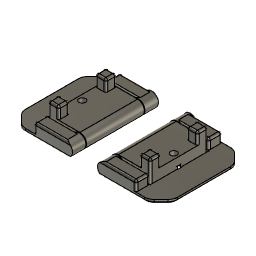
Voron-Simple-Hinge v20 (Autodesk Fusion 360 design; units mm, degrees)
Autodesk Fusion 360 part; units mm, degrees
note: some values were not read from the file. Set by a fixed rule: which sketch regions a step uses.
sketch "Sketch1" plane through (0, 0, 0) normal (0, 0, 1) x (1, 0, 0)
  circle A0 centre (0, 0) radius 1.6
  circle A1 centre (0, 0) radius 3.5
  line L0 (0, -3.5) -> (-16.5, -3.5)
  line L1 (-16.5, -3.5) -> (-16.5, 3.4)
  line L2 (-11, -3.5) -> (-11, -9.5)
  line L3 (-11, -9.5) -> (-16.5, -9.5)
  line L4 (-16.5, -9.5) -> (-16.5, -3.5)
  line L5 (-16.4, 3.5) -> (0, 3.5)
  arc A2 (-16.4, 3.5) -> (-16.5, 3.4) centre (-16.4, 3.4) ccw
  line L6 (-13.0173, 3.5) -> (-29.4, 3.5)
  line L7 (-29.5, 3.4) -> (-29.5, 1.5)
  line L8 (-29.5, 1.5) -> (-16.5, 1.5)
  arc A3 (-29.4, 3.5) -> (-29.5, 3.4) centre (-29.4, 3.4) ccw
  line L9 (-16.7917, 1.5) -> (-16.7917, 3.5)
  line L10 (0, 0) -> (-16.7917, 3.4812) construction
  line L11 (0, 0) -> (-16.7917, 2.5) construction
  line L12 (-3.5, 3.5) -> (-3.5, -3.5) construction
  line L13 (-29.5, 2.5) -> (-28.5, 3.5)
  line L14 (-16.5, 2.5) -> (-15.3897, 3.6103)
  line L15 (1.4497, 3.5) -> (2.4749, 2.4749)
  line L16 (0, 3.5) -> (1.4497, 3.5)
  point P0 (-16.5, 4.25)
  point P1 (-16.4979, 3.4203)
  dimension "d1" = 3.2
  dimension "d2" = 7
  dimension "d5" = 5.5
  dimension "d6" = 6
  dimension "d18" = 0.1
  dimension "d20" = 5
  dimension "d21" = 13
  dimension "d22" = 0.1
  dimension "d25" = 0.3
  dimension "d63" = 13
  dimension "d81" = 45
  dimension "d82" = 45
  dimension "d83" = 1
  dimension "d84" = 45
  constraint coincident A0.centre A1.centre
  constraint concentric A0 A1
  constraint horizontal L0
  constraint vertical L1
  constraint coincident A1 L0.start
  constraint tangent A1 L0
  constraint vertical L2
  constraint horizontal L3
  constraint vertical L4
  constraint coincident P0 L1
  constraint coincident A1 L5.end
  constraint tangent A1 L5
  constraint tangent L5 A2
  constraint tangent L1 A2
  constraint horizontal L5
  constraint horizontal L6
  constraint vertical L7
  constraint horizontal L8
  constraint coincident L5 L6.start
  constraint tangent L6 A3
  constraint tangent L7 A3
  constraint coincident L1 L8.end
  constraint coincident L8 L9.start
  constraint coincident L6 L9.end
  constraint perpendicular L6 L9
  constraint coincident L9 L10.end
  constraint coincident A2.centre L10
  constraint coincident A2 P1
  constraint coincident L10 P1
  constraint midpoint L9 L11.end
  constraint coincident L0 L2.start
  constraint coincident L5 L12.start
  constraint coincident L0 L12.end
  constraint perpendicular L0 L12
  constraint tangent A1 L12
  constraint coincident L7 L13.start
  constraint coincident L6 L13.end
  constraint coincident L1 L14.start
  constraint horizontal L13.start L14.start
  constraint coincident A1 L15.end
  constraint tangent A1 L15
  constraint coincident L15 L16.end
  constraint tangent A1 L16
  constraint coincident L15.start L16.end
  measures "d1" diameter of A0
  measures "d2" diameter of A1
  measures "d5" distance of L2.end L3.end
  measures "d6" distance of L0.end L3.end
  measures "d18" radius of A2
  measures "d20" distance of L0 L8
  measures "d21" distance of L1 L7
  measures "d22" radius of A3
  measures "d25" distance of L10.end P1
  measures "d63" distance of L1 L12
  measures "d81" angle of L7 L13
  measures "d82" angle of L1 L14
  measures "d83" distance of L6 L13.start
  measures "d84" angle of L15 L16
sketch "Sketch3" plane through (0, 0, 0) normal (0, 0, 1) x (1, 0, 0)
  circle A0 centre (0, 0) radius 2.35
  circle A1 centre (0, 0) radius 3.5
  dimension "d78" = 4.7
  constraint coincident A0.centre A1.centre
  measures "d78" diameter of A0
extrude "Extrude1" add sketch "Sketch1" along normal blind 5.5 contours A1 | A1 L15 L16 | A1 L0 L1 L5 L6 L14 | L0 L2 L3 L4 makes body 1
extrude "Extrude2" add sketch "Sketch1" along normal blind 19 from surface at 5.5 contours A1 | A1 L15 L16 | A1 L0 L1 L5 L6 L14 bodies 1
extrude "Extrude3" add sketch "Sketch1" along normal blind 5.5 from surface at 24.5 contours A1 | A1 L15 L16 | A1 L0 L1 L5 L6 L14 | L0 L2 L3 L4 bodies 1
extrude "Extrude4" add sketch "Sketch1" against normal blind 7 from surface at -0.3 separate body contours A0 | A1 | A1 L15 L16 | A1 L0 L1 L5 L6 L14 | L1 L5 A2 L6 L14 | L1 A2 L6 L8 L9 | L6 L7 L8 L9 L13 makes body 2
extrude "Extrude15" cut sketch "Sketch3" against normal up to surface (4.3 mm away) contours A0 bodies 2
extrude "Extrude5" add sketch "Sketch1" along normal up to surface (30.6 mm away) from surface at -0.3 contours L6 L7 L8 L9 L13 bodies 2
extrude "Extrude6" add sketch "Sketch1" along normal blind 7 from surface at 30.3 contours A1 | A1 L15 L16 | A1 L0 L1 L5 L6 L14 | L1 L5 A2 L6 L14 | L1 A2 L6 L8 L9 | L6 L7 L8 L9 L13 bodies 2
sketch "Sketch2" plane through (0, -3.5, 0) normal (0, -1, 0) x (1, 0, 0)
  line L0 (-11, 0) -> (0, 0)
  line L1 (0, 0) -> (0, 30)
  line L2 (0, 30) -> (-11, 30)
  line L3 (-11, 30) -> (-11, 24.5)
  line L4 (-11, 24.5) -> (-16.5, 24.5)
  line L5 (-16.5, 24.5) -> (-16.5, 5.5)
  line L6 (-16.5, 5.5) -> (-11, 5.5)
  line L7 (-11, 5.5) -> (-11, 0)
  line L8 (-13.75, 24.5) -> (-13.75, 5.5) construction
  circle A0 centre (-13.75, 15) radius 1.7
  circle A1 centre (-13.75, 15) radius 2.85
  line L9 (-29.5, 37.3) -> (-29.5, -7.3)
  line L10 (-29.5, -7.3) -> (-16.5, -7.3)
  line L11 (-16.5, -7.3) -> (-16.5, -0.3)
  line L12 (-16.5, -0.3) -> (-16.7917, -0.3)
  line L13 (-16.7917, -0.3) -> (-16.7917, 30.3)
  line L14 (-16.7917, 30.3) -> (-16.5, 30.3)
  line L15 (-16.5, 30.3) -> (-16.5, 37.3)
  line L16 (-16.5, 37.3) -> (-29.5, 37.3)
  line L17 (-23, 37.3) -> (-29.5, 30.8)
  line L18 (-13.75, 15) -> (-29.5, 15) construction
  line L19 (-23, -7.3) -> (-29.5, -0.8)
  circle A2 centre (-13.75, 15) radius 3.35
  dimension "d35" = 3.4
  dimension "d36" = 5.7
  dimension "d38" = 45
  dimension "d61" = 0.5
  constraint midpoint L4 L8.start
  constraint midpoint L6 L8.end
  constraint midpoint L8 A0.centre
  constraint concentric A0 A1
  constraint coincident L16 L17.start
  constraint coincident L9 L17.end
  constraint coincident A0.centre A1.centre
  constraint midpoint L9 L18.end
  constraint midpoint L16 L17.start
  constraint symmetric L17.start L18 L19.start
  constraint symmetric L17.end L18 L19.end
  measures "d35" diameter of A0
  measures "d36" diameter of A1
  measures "d38" angle of L16 L17
extrude "Extrude7" cut sketch "Sketch2" against normal through all contours L9 L10 L19 | L9 L16 L17 bodies 2
extrude "Extrude8" cut sketch "Sketch2" against normal through all contours A0 bodies 1
extrude "Extrude9" cut sketch "Sketch2" against normal up to surface (3 mm away) from surface at -4 contours L5 A1 L13 A2 | L5 A1 | L5 A1 bodies 2 1
extrude "Extrude12" cut sketch "Sketch2" against normal through all contours L13 A2 bodies 2
fillet "Fillet1" radius 1 26 edges at (-16.5, -3.5, 30) (-11, -6.5, 30) (-16.5, -6.5, 24.5) (-11, -6.5, 24.5) (-16.5, -6.5, 5.5) (-16.5, -3.5, 0) (-11, -6.5, 0) (-11, -6.5, 5.5) (-11, -9.5, 2.75) (-13.75, -9.5, 5.5) (-16.5, -9.5, 2.75) (-13.75, -9.5, 0) (-11, -9.5, 27.25) (-13.75, -9.5, 24.5) (-16.5, -9.5, 27.25) (-13.75, -9.5, 30) (-8.25, -3.5, 37.3) (-16.5, -3.5, 33.8) (-8.25, -3.5, 30.3) (-8.25, -3.5, -0.3) (-8.25, -3.5, -7.3) (-16.5, -3.5, -3.8) (-16.5, -1, 37.3) (-16.5, -1, 30.3) (-16.5, -1, -0.3) (-16.5, -1, -7.3) on bodies 1 2
fillet "Fillet2" radius 5 4 edges at (-29.5, 2, -0.8) (-23, 2.5, -7.3) (-23, 2.5, 37.3) (-29.5, 2, 30.8) on bodies 2
extrude "Extrude10" add sketch "Sketch1" along normal up to surface (7 mm away) from surface at 30.3 contours A1 bodies 2
chamfer "Chamfer2" distance 1 angle 45 8 edges at (-9.7396, 3.5, -7.3) (-28.2773, 3.5, -2.0049) (-26.25, 3.5, -4.05) (-22.8423, 3.5, -6.9194) (-9.7396, 3.5, 37.3) (-22.8423, 3.5, 36.9194) (-26.25, 3.5, 34.05) (-28.2773, 3.5, 32.0049) on bodies 2
extrude "Extrude11" add sketch "Sketch3" against normal up to surface (4 mm away) from surface at -0.3 bodies 2
chamfer "Chamfer1" distance 1.15 angle 45 1 edges at (-15.335, 0.5, 15.6147) on bodies 1
move_body "Move1" bodies 2 1 to x (1, 0, 0) y (0, 0, -1) z (0, 1, 0) at (0, -33.5, 26.5)
copy_body "Body->Comp1" bodies 1 removing the originals makes body 3 in component "Fixed Leaf Left"
copy_body "Body->Comp2" bodies 2 removing the originals makes body 4 in component "Moving Leaf Left"
ref_plane "WorkPlane1" through (10, 0, 0) normal (1, 0, 0) x (0, 1, 0)
mirror "MirrorComponent1" about plane through (0, 0, 0) normal (0, 0, 1) of bodies 4 makes body 5 in component "Moving Leaf Right"
mirror "MirrorComponent1'" about plane through (0, 0, 0) normal (0, 0, 1) of bodies 3 makes body 6 in component "Fixed Leaf Right"
component "Left" placed x (1, 0, 0) y (0, 1, 0) z (0, 0, 1) at (0, 0, 0)
component "Right" placed x (1, 0, 0) y (0, 1, 0) z (0, 0, 1) at (0, 0, 0)
component "Fixed Leaf Left" placed x (1, 0, 0) y (0, 1, 0) z (0, 0, 1) at (0, 0, 0) in component "Left"
component "Moving Leaf Left" placed x (1, 0, 0) y (0, 1, 0) z (0, 0, 1) at (0, 0, 0) in component "Left"
component "Fixed Leaf Right" placed x (-1, 0, 0) y (0, 1, 0) z (0, 0, -1) at (20, 0, 0) in component "Right"
component "Moving Leaf Right" placed x (-1, 0, 0) y (0, 1, 0) z (0, 0, -1) at (20, 0, 0) in component "Right"
equation "d1 = PinDiameter"
equation "d20 = PanelDepth"
equation "d25 = HingeGap"
equation "d26 = -HingeGap"
equation "d30 = HingeGap"
equation "d50 = 0 mm - HingeGap"
equation "d55 = -LowerMovingLeafPinClosure"
equation "HingeGap = 0.3 mm"
equation "d63 = 6 mm + 7 mm"
equation "PinDiameter = 3.2 mm" comment "3.2 for m3, 1.75 for filament"
equation "LowerMovingLeafPinDiameter = 4.7 mm" comment "4.7 for heat set, 1.75 for filament"
equation "LowerMovingLeafPinClosure = 3 mm" comment "Set to 1 for filament or 3 for heat set"
equation "PanelDepth = 5 mm" comment "Depth of front panel including foam"
equation "d78 = LowerMovingLeafPinDiameter"
equation "d79 = -LowerMovingLeafPinClosure"
